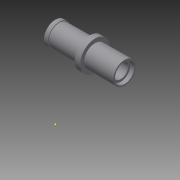
# Autodesk Inventor part: AxleTL
Saved by Autodesk Inventor 2015 (Build 190159000, 159)
## iProperties
Created: 2015-01-29
Part Number: AxleTL
Material: Generic
Document SubType Name: Modeling
Designer: PLTW-Stu-02
Density: 1 g/cm^3
Appearance: Default
Author: PLTW-Stu-02
Autodesk Inventor part; units mm, degrees
ref_plane "YZ Plane" through (0, 0, 0) normal (1, 0, 0) x (0, 1, 0)
ref_plane "XZ Plane" through (0, 0, 0) normal (0, 1, 0) x (-1, 0, 0)
sketch "Sketch1" plane through (0, 0, 0) normal (0, 0, 1) x (1, 0, 0)
  line L0 (56.5885, 25.8826) -> (56.5885, 28.2956)
  line L1 (56.5885, 28.2956) -> (64.9705, 28.2956)
  line L2 (64.9705, 28.2956) -> (64.9705, 29.0576)
  line L3 (64.9705, 29.0576) -> (66.2405, 29.0576)
  line L4 (66.2405, 29.0576) -> (66.2405, 29.5656)
  line L5 (54.153, 29.4566) -> (44.9045, 29.3732)
  line L6 (54.153, 29.4566) -> (54.8105, 29.4566) construction
  line L7 (56.5885, 30.7581) -> (54.8105, 30.7581)
  line L8 (66.2405, 29.5656) -> (56.5885, 29.4785)
  line L9 (54.8105, 29.4625) -> (54.153, 29.4566)
  line L10 (56.5885, 30.7581) -> (56.5885, 29.4785)
  line L11 (54.8105, 30.7581) -> (54.8105, 29.4625)
  line L12 (44.9045, 29.3732) -> (44.9045, 29.6272)
  line L13 (44.9045, 29.6272) -> (43.6345, 29.6272)
  line L14 (43.6345, 29.6272) -> (43.6345, 28.9922)
  line L15 (43.6345, 28.9922) -> (49.9845, 28.9922)
  line L16 (49.9845, 28.9922) -> (49.9845, 28.2302)
  line L17 (49.9845, 28.2302) -> (54.8105, 28.2302)
  line L18 (54.8105, 28.2302) -> (54.8105, 25.8826)
  line L19 (44.9045, 25.8826) -> (67.1022, 25.8826) construction
  line L20 (54.8105, 25.8826) -> (56.5885, 25.8826)
  point P0 (0, 0)
  constraints: 42 end point, 10 perpendicular, 3 horizontal, 3 vertical, 1 parallel
revolve "Revolution1" add sketch "Sketch1" angle 360 about axis through (44.9045, 25.8826, 0) along (1, 0, 0)
ref_plane "Work Plane1" through (43.6345, 25.8826, 0) normal (-1, 0, 0) x (0, 0, 1)
sketch "Sketch5" plane through (43.6345, 25.8826, 0) normal (-1, 0, 0) x (0, 0, 1)
  point P0 (0, -25.8826)
body "Solid1"
